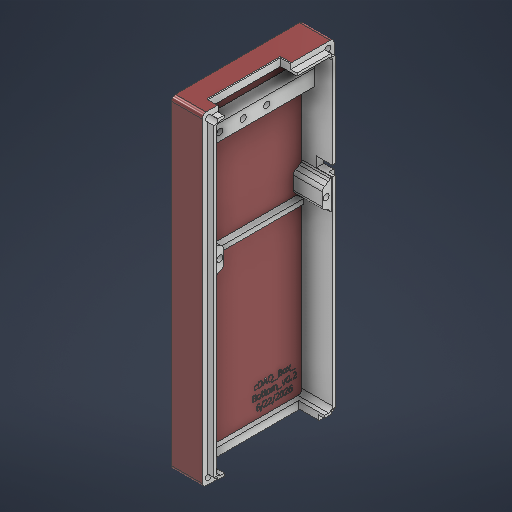
# Autodesk Inventor part: cDAQ_Box_Bottom_v0.2.2ipt
Saved by Autodesk Inventor 2027 (Build 310192000, 192)
## iProperties
Created: 2026-05-08
Part Number: cDAQ_Box_Bottom_v0.2.2ipt
Material: Generic
Document SubType Name: Modeling
Designer: giese
Density: 1 g/cm^3
Appearance: Default
Author: giese
Autodesk Inventor part; units mm, degrees
(part 1 of 2)
ref_plane "YZ Plane" through (0, 0, 0) normal (1, 0, 0) x (0, 1, 0)
ref_plane "XZ Plane" through (0, 0, 0) normal (0, 1, 0) x (-1, 0, 0)
ref_plane "XY Plane" through (0, 0, 0) normal (0, 0, 1) x (1, 0, 0)
sketch "Sketch1" plane through (0, 0, 0) normal (1, 0, 0) x (0, 1, 0)
  line L0 (37.5698, 55.7067) -> (-217.4462, 55.7067)
  line L1 (-217.4462, 55.7067) -> (-217.4462, -48.4333)
  line L2 (-217.4462, -48.4333) -> (37.5698, -48.4333)
  line L3 (37.5698, -48.4333) -> (37.5698, 55.7067)
  point P0 (0, 0)
  dimension "d0" = 104.14
  dimension "d1" = 255.016
  constraints: 8 end point, 2 parallel, 1 horizontal, 1 perpendicular
  measures "d0" distance of L2.end L0.start
  measures "d1" distance of L1.end L2.end
extrude "Extrusion1" add sketch "Sketch1" along normal blind 24.13
sketch "Sketch2" plane through (24.13, 0, 0) normal (1, 0, 0) x (0, 0, -1)
  line L0 (42.0833, 31.2198) -> (-49.3567, 31.2198)
  line L1 (-49.3567, 31.2198) -> (-49.3567, -211.0962)
  line L2 (-49.3567, -211.0962) -> (42.0833, -211.0962)
  line L3 (42.0833, -211.0962) -> (42.0833, 31.2198)
  line L4 (48.4333, 37.5698) -> (-55.7067, 37.5698) projected
  line L5 (-55.7067, 37.5698) -> (-55.7067, -217.4462) projected
  line L6 (-55.7067, -217.4462) -> (48.4333, -217.4462) projected
  line L7 (48.4333, -217.4462) -> (48.4333, 37.5698) projected
  point P0 (0, 0)
  dimension "d4" = 242.316
  dimension "d5" = 91.44
  dimension "d8" = 6.35
  dimension "d21" = 6.35
  dimension "d690" = 6.35
  dimension "d842" = 6.35
  constraints: 8 end point, 2 parallel, 1 horizontal, 1 perpendicular
  measures "d4" distance of L2.end L0.start
  measures "d5" distance of L0.start L0.end
  measures "d8" distance between parallel lines of L0 L4
  measures "d21" distance between parallel lines of L5 L1
  measures "d690" distance between parallel lines of L6 L2
  measures "d842" distance between parallel lines of L7 L3
extrude "Extrusion2" cut sketch "Sketch2" against normal blind 19.05 contours L3 L2 L1 L0
sketch "Sketch3" plane through (0, 0, 0) normal (-1, 0, 0) x (0, 0, 1)
  circle A0 centre (-4.1509, 9.6298) radius 2.4005
  circle A1 centre (14.3479, 9.6298) radius 2.4005
  circle A2 centre (32.8467, 9.6298) radius 2.4005
  line L0 (-48.4333, -217.4462) -> (-48.4333, 37.5698) projected
  line L1 (-48.4333, 37.5698) -> (55.7067, 37.5698) projected
  line L2 (55.7067, 37.5698) -> (55.7067, -217.4462) projected
  line L3 (49.3567, 31.2198) -> (-42.0833, 31.2198) projected
  point P0 (0, 0)
  point P1 (-0.896, -23.7433)
  point P2 (-45.1848, 27.0137)
  dimension "d9" = 18.4988
  dimension "d10" = 4.801
  dimension "d11" = 4.801
  dimension "d12" = 18.4988
  dimension "d13" = 36.9976
  dimension "d18" = 22.86
  dimension "d22" = 4.801
  dimension "d58" = 27.94
  constraints: 3 centre point
  measures "d9" distance of A0.centre A1.centre
  measures "d10" diameter of A1
  measures "d11" diameter of A2
  measures "d12" distance of A1.centre A2.centre
  measures "d13" distance of A0.centre A2.centre
  measures "d18" distance from line of L2 A2.centre
  measures "d22" diameter of A0
  measures "d58" distance from line of L1 A2.centre
extrude "Extrusion3" cut sketch "Sketch3" against normal blind 5.08
sketch "Sketch5" plane through (0, -217.4462, -48.4333) normal (0, 0, -1) x (-1, 0, 0)
  line L0 (-27.2034, 165.862) -> (-16.51, 165.862)
  line L1 (-16.51, 165.862) -> (-16.51, 173.862)
  line L2 (-16.51, 173.862) -> (-27.2034, 173.862)
  line L3 (-27.2034, 173.862) -> (-27.2034, 165.862)
  line L4 (0, 255.016) -> (-24.13, 255.016) projected
  line L5 (0, 0) -> (0, 255.016) projected
  line L6 (-24.13, 0) -> (-24.13, 255.016) projected
  line L7 (0, 0) -> (-24.13, 0) projected
  point P0 (0, 217.4462)
  point P1 (-21.8567, 173.862)
  point P2 (-21.8567, 165.862)
  dimension "d28" = 10.6934
  dimension "d30" = 8
  dimension "d31" = 16.51
  dimension "d215" = 3.0734
  dimension "d1133" = 165.862
  constraints: 8 end point, 2 midpoint, 2 parallel, 1 horizontal, 1 perpendicular
  measures "d28" distance between parallel lines of L1 L3
  measures "d30" distance of point (-21.857, 173.862) point (-21.857, 165.862)
  measures "d31" distance between parallel lines of L5 L1
  measures "d215" distance between parallel lines of L6 L3
  measures "d1133" distance between parallel lines of L7 L0
extrude "Extrusion4" cut sketch "Sketch5" against normal blind 24.13 contours L3 L2 L6 L0 | L6 L2 L1 L0
sketch "Sketch6" plane through (0, -217.4462, -48.4333) normal (0, -1, 0) x (1, 0, 0)
  line L0 (24.08, 55.136) -> (16.08, 55.136)
  line L1 (16.08, 45.136) -> (24.08, 45.136)
  line L2 (0, 104.14) -> (0, 0) projected
  line L3 (29.63, 53.1359) -> (29.63, 47.136)
  line L4 (24.08, 55.136) -> (29.63, 53.1359)
  line L5 (29.63, 47.136) -> (24.08, 45.136)
  line L6 (0, 0) -> (24.13, 0) projected
  line L7 (24.13, 97.79) -> (24.13, 6.35) projected
  line L8 (24.13, 41.9134) -> (24.13, 37.4697)
  line L9 (16.08, 55.136) -> (8.636, 55.136)
  line L10 (8.636, 55.136) -> (8.636, 45.136)
  line L11 (8.636, 45.136) -> (21.16, 45.136)
  point P0 (0, 48.4333)
  point P1 (20.08, 55.136)
  point P2 (20.08, 45.136)
  point P3 (16.08, 50.136)
  dimension "d39" = 6
  dimension "d48" = 55.136
  dimension "d221" = 0
  dimension "d223" = 2
  dimension "d224" = 2
  dimension "d225" = 5.5
  dimension "d227" = 5.55
  dimension "d672" = 8.636
  constraints: 18 end point, 2 horizontal, 2 midpoint, 2 parallel, 2 point on line, 1 perpendicular, 1 vertical
  measures "d39" distance of L3.start L3.end
  measures "d48" distance between parallel lines of L6 L0
  measures "d221" horizontal distance of L0.start L1.end
  measures "d223" vertical distance of L3.end L1.end
  measures "d224" vertical distance of L0.start L3.start
  measures "d225" distance between parallel lines of L3 L7
  measures "d227" distance from line of L1.end L3
  measures "d672" distance between parallel lines of L2 L10
extrude "Extrusion5" [suppressed]
sketch "Sketch7" plane through (0, 37.5698, 55.7067) normal (0, 1, 0) x (1, 0, 0)
  line L0 (31.0134, 69.85) -> (16.002, 69.85)
  line L1 (16.002, 69.85) -> (16.002, 12.7)
  line L2 (16.002, 12.7) -> (31.0134, 12.7)
  line L3 (31.0134, 12.7) -> (31.0134, 69.85)
  line L4 (0, 0) -> (24.13, 0) projected
  line L5 (0, 104.14) -> (0, 0) projected
  line L6 (24.13, 104.14) -> (24.13, 0) projected
  point P0 (0, 55.7067)
  point P1 (24.13, 69.85)
  point P2 (24.13, 12.7)
  dimension "d52" = 12.7
  dimension "d55" = 16.002
  dimension "d56" = 15.0114
  dimension "d57" = 6.8834
  dimension "d1195" = 69.85
  constraints: 8 end point, 2 parallel, 1 horizontal, 1 perpendicular
  measures "d52" distance between parallel lines of L4 L2
  measures "d55" distance between parallel lines of L5 L1
  measures "d56" distance between parallel lines of L3 L1
  measures "d57" distance between parallel lines of L6 L3
  measures "d1195" distance between parallel lines of L4 L0
extrude "Extrusion6" cut sketch "Sketch7" against normal blind 7.62
fillet "Fillet1" radius 3.175 4 edges at (12.065, 37.5698, -48.4333) (12.065, 37.5698, 55.7067) (12.065, -217.4462, -48.4333) (12.065, -217.4462, 55.7067)
sketch "Sketch8" plane through (0, 0, 0) normal (-1, 0, 0) x (0, 0, 1)
  line L0 (-5.9225, 6.0992) -> (-2.3919, 6.0992)
  line L1 (-5.9225, 13.1604) -> (-2.3919, 13.1604)
  line L2 (-5.9225, 6.0992) -> (-7.9609, 9.6298)
  line L3 (-5.9225, 13.1604) -> (-7.9609, 9.6298)
  line L4 (-2.3919, 6.0992) -> (-0.3536, 9.6298)
  line L5 (-2.3919, 13.1604) -> (-0.3536, 9.6298)
  circle A0 centre (-4.1509, 9.6298) radius 2.4005 projected
  line L6 (12.5763, 6.0992) -> (16.1069, 6.0992)
  line L7 (12.5763, 13.1604) -> (16.1069, 13.1604)
  line L8 (12.5763, 6.0992) -> (10.5379, 9.6298)
  line L9 (12.5763, 13.1604) -> (10.5379, 9.6298)
  line L10 (16.1069, 6.0992) -> (18.1453, 9.6298)
  line L11 (16.1069, 13.1604) -> (18.1453, 9.6298)
  circle A1 centre (14.3479, 9.6298) radius 2.4005 projected
  line L12 (31.0751, 6.0992) -> (29.0367, 9.6298)
  line L13 (31.0751, 13.1604) -> (29.0367, 9.6298)
  line L14 (31.0751, 6.0992) -> (34.6057, 6.0992)
  line L15 (31.0751, 13.1604) -> (34.6057, 13.1604)
  line L16 (34.6057, 6.0992) -> (36.6441, 9.6298)
  line L17 (34.6057, 13.1604) -> (36.6441, 9.6298)
  circle A2 centre (32.8467, 9.6298) radius 2.4005 projected
  point P0 (-4.1572, 6.0992)
  point P1 (14.3416, 6.0992)
  point P2 (32.8404, 6.0992)
  point P3 (-7.9609, 9.6298)
  point P4 (-0.3536, 9.6298)
  point P5 (18.1453, 9.6298)
  point P6 (10.5379, 9.6298)
  point P7 (36.6441, 9.6298)
  point P8 (29.0367, 9.6298)
  dimension "d60" = 7.0612
  dimension "d61" = 120
  dimension "d62" = 120
  dimension "d63" = 120
  dimension "d64" = 120
  dimension "d65" = 3.5306
  dimension "d66" = 3.5306
  dimension "d67" = 3.5306
  dimension "d68" = 3.5306
  dimension "d69" = 3.5306
  dimension "d70" = 3.5306
  dimension "d71" = 0
  dimension "d72" = 7.6074
  dimension "d73" = 3.81
  dimension "d74" = 0
  dimension "d75" = 7.0612
  dimension "d76" = 120
  dimension "d77" = 120
  dimension "d78" = 120
  dimension "d79" = 120
  dimension "d80" = 3.5306
  dimension "d81" = 3.5306
  dimension "d82" = 3.5306
  dimension "d83" = 3.5306
  dimension "d84" = 3.5306
  dimension "d85" = 3.5306
  dimension "d86" = 0
  dimension "d87" = 7.6074
  dimension "d91" = 0
  dimension "d92" = 3.81
  dimension "d93" = 7.0612
  dimension "d94" = 120
  dimension "d95" = 120
  dimension "d96" = 120
  dimension "d97" = 120
  dimension "d98" = 3.5306
  dimension "d99" = 3.5306
  dimension "d100" = 3.5306
  dimension "d101" = 3.5306
  dimension "d102" = 3.5306
  dimension "d103" = 3.5306
  dimension "d104" = 0
  dimension "d105" = 7.6074
  dimension "d108" = 0
  dimension "d109" = 3.81
  constraints: 36 end point, 6 horizontal, 3 midpoint
  measures "d60" distance from line of point (-4.157, 6.099) L1
  measures "d61" angle of L0 L2
  measures "d62" angle of L1 L3
  measures "d63" angle of L4 L0
  measures "d64" angle of L5 L1
  measures "d65" distance of L0.start L0.end
  measures "d66" distance of L1.start L1.end
  measures "d67" vertical distance of L1.start L3.end
  measures "d68" vertical distance of L0.start L2.end
  measures "d69" vertical distance of L1.end L5.end
  measures "d70" vertical distance of L0.end L4.end
  measures "d71" horizontal distance of L0.start L1.start
  measures "d72" distance of L4.end L2.end
  measures "d73" distance of A0.centre L2.end
  measures "d74" vertical distance of A0.centre L4.end
  measures "d75" distance from line of point (14.342, 6.099) L7
  measures "d76" angle of L6 L8
  measures "d77" angle of L7 L9
  measures "d78" angle of L10 L6
  measures "d79" angle of L11 L7
  measures "d80" distance of L8.start L6.end
  measures "d81" distance of L9.start L7.end
  measures "d82" vertical distance of L9.start L9.end
  measures "d83" vertical distance of L8.start L8.end
  measures "d84" vertical distance of L7.end L11.end
  measures "d85" vertical distance of L6.end L10.end
  measures "d86" horizontal distance of L8.start L9.start
  measures "d87" distance of L10.end L8.end
  measures "d91" vertical distance of A1.centre L8.end
  measures "d92" distance of A1.centre L8.end
  measures "d93" distance from line of point (32.84, 6.099) L15
  measures "d94" angle of L14 L12
  measures "d95" angle of L15 L13
  measures "d96" angle of L16 L14
  measures "d97" angle of L17 L15
  measures "d98" distance of L12.start L16.start
  measures "d99" distance of L15.start L15.end
  measures "d100" vertical distance of L15.start L13.end
  measures "d101" vertical distance of L12.start L12.end
  measures "d102" vertical distance of L15.end L17.end
  measures "d103" vertical distance of L16.start L16.end
  measures "d104" horizontal distance of L12.start L15.start
  measures "d105" distance of L16.end L12.end
  measures "d108" vertical distance of A2.centre L12.end
  measures "d109" distance of A2.centre L12.end
extrude "Extrusion7" cut sketch "Sketch8" against normal blind 4 contours L2 L3 L1 L5 L4 L0 | A0 | L8 L9 L7 L11 L10 L6 | A1 | L12 L13 L15 L17 L16 L14 | A2
sketch "Sketch9" plane through (5.08, 0, 0) normal (1, 0, 0) x (0, 0, -1)
  arc A0 (24.8089, -180.8044) -> (19.3527, -180.8044) centre (22.0808, -178.3302) ccw
  line L0 (45.2583, 37.5698) -> (14.1433, 37.5698) projected
  line L1 (42.0833, 31.2198) -> (42.0833, -43.5842) projected
  arc A1 (20.1758, -185.9502) -> (23.9858, -185.9502) centre (22.0808, -185.9502) ccw
  line L2 (23.9858, -185.9502) -> (23.9858, -182.9374)
  line L3 (20.1758, -185.9502) -> (20.1758, -182.9374)
  arc A2 (24.8089, -180.8044) -> (23.9858, -182.9374) centre (27.1608, -182.9374) ccw
  arc A3 (20.1758, -182.9374) -> (19.3527, -180.8044) centre (17.0008, -182.9374) ccw
  arc A4 (-25.9911, -180.8044) -> (-31.4473, -180.8045) centre (-28.7192, -178.3302) ccw
  arc A5 (-30.6242, -185.9366) -> (-26.8142, -185.9502) centre (-28.7192, -185.9502) ccw
  line L4 (-26.8142, -185.9502) -> (-26.8142, -182.9374)
  line L5 (-30.6242, -185.9366) -> (-30.6242, -182.9374)
  arc A6 (-25.9911, -180.8044) -> (-26.8142, -182.9374) centre (-23.6392, -182.9374) ccw
  arc A7 (-30.6242, -182.9374) -> (-31.4473, -180.8045) centre (-33.7992, -182.9374) ccw
  line L6 (-43.0067, 37.5698) -> (-52.5317, 37.5698) projected
  line L7 (-49.3567, -211.0962) -> (-49.3567, 31.2198) projected
  point P0 (0, 0)
  point P1 (42.0833, -211.0962)
  point P2 (23.9858, -181.4823)
  point P3 (20.1758, -181.4823)
  point P4 (-26.8142, -181.4823)
  point P5 (-30.6242, -181.4823)
  point P6 (-49.3567, 31.2198)
  point P7 (-46.8167, -217.4462)
  dimension "d112" = 215.9
  dimension "d114" = 7.366
  dimension "d116" = 3.81
  dimension "d117" = 223.52
  dimension "d118" = 3.175
  dimension "d119" = 7.366
  dimension "d120" = 3.81
  dimension "d121" = 3.175
  dimension "d122" = 215.9
  dimension "d123" = 223.52
  dimension "d125" = 0
  dimension "d128" = 50.8
  dimension "d129" = 20.0025
  dimension "d130" = 0
  constraints: 20 point on circle, 8 centre point, 8 end point, 8 tangent, 4 point on line, 2 equal radius, 2 parallel, 2 vertical, 1 other
  measures "d112" distance from line of L0 A0.centre
  measures "d114" diameter of A0
  measures "d116" diameter of A1
  measures "d117" distance from line of L0 A1.centre
  measures "d118" radius of A2
  measures "d119" diameter of A4
  measures "d120" diameter of A5
  measures "d121" radius of A6
  measures "d122" distance from line of A4.centre L6
  measures "d123" distance from line of L6 A5.centre
  measures "d125" horizontal distance of A5.centre A4.centre
  measures "d128" distance of A5.centre A1.centre
  measures "d129" distance from line of L1 A0.centre
  measures "d130" horizontal distance of A0.centre A1.centre
extrude "Extrusion8" [suppressed]
sketch "Sketch10" plane through (24.13, 0, 0) normal (1, 0, 0) x (0, 0, -1)
  line L0 (-49.3567, 31.2198) -> (42.0833, 31.2198) projected
  line L1 (-49.3567, 31.2198) -> (42.0833, 31.2198)
  line L2 (42.0833, 33.2264) -> (-46.8167, 33.2264)
  line L3 (-46.8167, 33.2264) -> (-51.3633, 33.2264)
  line L4 (-51.3633, 33.2264) -> (-51.3633, -213.1028)
  line L5 (-51.3633, -213.1028) -> (44.0899, -213.1028)
  line L6 (44.0899, -213.1028) -> (44.0899, 33.2264)
  line L7 (44.0899, 33.2264) -> (41.9392, 33.2264)
  line L8 (42.0833, 31.2198) -> (42.0833, -43.5842) projected
  line L9 (-49.3567, -211.0962) -> (-49.3567, 31.2198) projected
  line L10 (42.0833, -211.0962) -> (-49.3567, -211.0962) projected
  line L11 (45.2583, 37.5698) -> (14.1433, 37.5698) projected
  line L12 (42.0833, 31.2198) -> (42.0833, -211.0962)
  line L13 (42.0833, -211.0962) -> (-49.3567, -211.0962)
  line L14 (-52.5317, -217.4462) -> (45.2583, -217.4462) projected
  line L15 (-49.3567, -211.0962) -> (-49.3567, 31.2198)
  line L16 (-49.3567, 31.2198) -> (42.0833, 31.2198)
  point P0 (-46.8167, -217.4462)
  dimension "d202" = 2.0066
  dimension "d203" = 2.0066
  dimension "d204" = 2.0066
  dimension "d205" = 2.0066
  dimension "d208" = 4.3434
  constraints: 22 end point, 5 perpendicular, 3 point on line, 2 parallel, 1 collinear, 1 horizontal, 1 other
  measures "d202" distance between parallel lines of L0 L2
  measures "d203" distance between parallel lines of L6 L8
  measures "d205" distance between parallel lines of L5 L10
  measures "d208" distance between parallel lines of L11 L2
extrude "Extrusion9" add sketch "Sketch10" along normal blind 5
fillet "Fillet2" radius 3.175 8 edges at (17.105, 31.2198, -42.0833) (17.105, 31.2198, 49.3567) (17.105, -211.0962, 49.3567) (17.105, -211.0962, -42.0833) (26.63, 33.2264, -44.0899) (26.63, 33.2264, 51.3633) (26.63, -213.1028, -44.0899) (26.63, -213.1028, 51.3633)
sketch "Sketch13" plane through (29.13, 0, 0) normal (1, 0, 0) x (0, 0, -1)
  arc A0 (44.0833, 30.0448) -> (40.9083, 33.2198) centre (40.9083, 30.0448) ccw projected
  arc A1 (-45.6417, 33.2198) -> (-48.8167, 30.0448) centre (-45.6417, 30.0448) ccw projected
  arc A2 (40.9083, -212.0802) -> (44.0833, -208.9052) centre (40.9083, -208.9052) ccw projected
  arc A3 (-48.8167, -208.9052) -> (-45.6417, -212.0802) centre (-45.6417, -208.9052) ccw projected
  line L0 (-43.0067, 37.5698) -> (-52.5317, 37.5698) projected
  line L1 (-55.7067, 34.3948) -> (-55.7067, -214.2712) projected
  line L2 (-52.5317, -217.4462) -> (45.2583, -217.4462) projected
  arc A4 (-48.8167, -208.9052) -> (-45.6417, -212.0802) centre (-45.6417, -208.9052) ccw projected
  circle A5 centre (-50.6267, -212.3662) radius 2.4005
  circle A6 centre (43.3533, -212.3662) radius 2.4005
  line L3 (48.4333, -214.2712) -> (48.4333, 34.3948) projected
  circle A7 centre (43.3533, 32.4898) radius 2.4005
  line L4 (45.2583, 37.5698) -> (14.1433, 37.5698) projected
  circle A8 centre (-50.6267, 32.4898) radius 2.4005
  arc A9 (41.4904, -28.6131) -> (38.3154, -25.4381) centre (38.3154, -28.6131) ccw
  circle A10 centre (38.2733, -64.0302) radius 2.4005
  circle A11 centre (-45.5467, -64.0302) radius 2.4005
  point P0 (0, 0)
  point P1 (-47.8868, 32.2898)
  point P2 (-47.8868, -211.1503)
  point P3 (-47.8868, -211.1503)
  point P4 (45.8404, -24.2631)
  point P5 (42.6654, -21.0881)
  dimension "d178" = 5.08
  dimension "d179" = 5.08
  dimension "d180" = 4.801
  dimension "d181" = 5.08
  dimension "d182" = 5.08
  dimension "d183" = 4.801
  dimension "d184" = 4.801
  dimension "d185" = 5.08
  dimension "d186" = 5.08
  dimension "d187" = 4.801
  dimension "d188" = 5.08
  dimension "d189" = 5.08
  dimension "d326" = 4.801
  dimension "d327" = 10.16
  dimension "d328" = 101.6
  dimension "d329" = 4.801
  dimension "d330" = 10.16
  dimension "d331" = 101.6
  constraints: 7 centre point, 5 point on circle
  measures "d178" distance from line of L1 A5.centre
  measures "d179" distance from line of L2 A5.centre
  measures "d180" diameter of A5
  measures "d181" distance from line of L2 A6.centre
  measures "d182" distance from line of L3 A6.centre
  measures "d183" diameter of A6
  measures "d184" diameter of A7
  measures "d185" distance from line of L3 A7.centre
  measures "d186" distance from line of L4 A7.centre
  measures "d187" diameter of A8
  measures "d188" distance from line of L0 A8.centre
  measures "d189" distance from line of L1 A8.centre
  measures "d326" diameter of A10
  measures "d327" distance from line of L3 A10.centre
  measures "d328" distance from line of A10.centre L4
  measures "d329" diameter of A11
  measures "d330" distance from line of L1 A11.centre
  measures "d331" distance from line of L0 A11.centre
extrude "Extrusion11" cut sketch "Sketch13" against normal blind 25.4
sketch "Sketch14" plane through (5.08, 0, 0) normal (1, 0, 0) x (0, 0, -1)
  line L0 (10.8408, -186.2545) -> (30.0575, -186.2545) construction
  line L1 (30.0575, -186.2545) -> (30.0575, -184.305) construction
  line L2 (30.0575, -184.305) -> (10.8408, -184.305) construction
  line L3 (10.8408, -184.305) -> (10.8408, -186.2545) construction
  spline S0 degree 2 poles (5.944, -191.0006) (5.5883, -191.0006) (4.9992, -190.782) (4.788, -190.5597) knots 0 0 0 1 2 2 2
  spline S1 degree 2 poles (4.788, -190.5597) (4.5768, -190.3411) (4.3434, -189.6668) (4.3434, -189.2148) knots 0 0 0 1 2 2 2
  spline S2 degree 2 poles (4.3434, -189.2148) (4.3434, -188.7628) (4.5842, -188.1033) (4.788, -187.881) knots 0 0 0 1 2 2 2
  spline S3 degree 2 poles (4.788, -187.881) (4.9918, -187.655) (5.5957, -187.4141) (5.944, -187.4141) knots 0 0 0 1 2 2 2
  spline S4 degree 2 poles (5.944, -187.4141) (6.2255, -187.4141) (6.7517, -187.5735) (6.9554, -187.6772) knots 0 0 0 1 2 2 2
  line L4 (6.9554, -187.6772) -> (6.9554, -188.3256)
  line L5 (6.9554, -188.3256) -> (6.9221, -188.3256)
  spline S5 degree 2 poles (6.9221, -188.3256) (6.8591, -188.2737) (6.6664, -188.1403) (6.5294, -188.0699) knots 0 0 0 1 2 2 2
  spline S6 degree 2 poles (6.5294, -188.0699) (6.4071, -188.0106) (6.081, -187.918) (5.9328, -187.918) knots 0 0 0 1 2 2 2
  spline S7 degree 2 poles (5.9328, -187.918) (5.4845, -187.918) (4.9399, -188.596) (4.9399, -189.2148) knots 0 0 0 1 2 2 2
  spline S8 degree 2 poles (4.9399, -189.2148) (4.9399, -189.8187) (5.466, -190.4967) (5.9328, -190.4967) knots 0 0 0 1 2 2 2
  spline S9 degree 2 poles (5.9328, -190.4967) (6.2144, -190.4967) (6.7257, -190.2633) (6.9221, -190.0818) knots 0 0 0 1 2 2 2
  line L6 (6.9221, -190.0818) -> (6.9554, -190.0818)
  line L7 (6.9554, -190.0818) -> (6.9554, -190.7301)
  spline S10 degree 2 poles (6.9554, -190.7301) (6.8702, -190.7709) (6.6109, -190.8857) (6.5071, -190.9117) knots 0 0 0 1 2 2 2
  spline S11 degree 2 poles (6.5071, -190.9117) (6.3589, -190.9561) (6.1255, -191.0006) (5.944, -191.0006) knots 0 0 0 1 2 2 2
  spline S12 degree 2 poles (11.131, -188.6405) (11.131, -189.2666) (10.6234, -190.2744) (10.1973, -190.556) knots 0 0 0 1 2 2 2
  spline S13 degree 2 poles (10.1973, -190.556) (9.8491, -190.7746) (9.134, -190.9228) (8.5782, -190.9228) knots 0 0 0 1 2 2 2
  line L8 (8.5782, -190.9228) -> (7.526, -190.9228)
  line L9 (7.526, -190.9228) -> (7.526, -186.3508)
  line L10 (7.526, -186.3508) -> (8.5671, -186.3508)
  spline S14 degree 2 poles (8.5671, -186.3508) (9.2118, -186.3508) (9.9454, -186.5435) (10.2047, -186.7139) knots 0 0 0 1 2 2 2
  spline S15 degree 2 poles (10.2047, -186.7139) (10.6456, -187.0066) (11.131, -187.9736) (11.131, -188.6405) knots 0 0 0 1 2 2 2
  spline S16 degree 2 poles (10.4974, -188.6331) (10.4974, -188.107) (10.1492, -187.3623) (9.8046, -187.1511) knots 0 0 0 1 2 2 2
  spline S17 degree 2 poles (9.8046, -187.1511) (9.5601, -187.0066) (9.008, -186.8769) (8.5968, -186.8769) knots 0 0 0 1 2 2 2
  line L11 (8.5968, -186.8769) -> (8.1336, -186.8769)
  line L12 (8.1336, -186.8769) -> (8.1336, -190.3967)
  line L13 (8.1336, -190.3967) -> (8.5968, -190.3967)
  spline S18 degree 2 poles (8.5968, -190.3967) (9.0006, -190.3967) (9.6119, -190.267) (9.8602, -190.0929) knots 0 0 0 1 2 2 2
  spline S19 degree 2 poles (9.8602, -190.0929) (10.1788, -189.878) (10.4974, -189.1666) (10.4974, -188.6331) knots 0 0 0 1 2 2 2
  line L14 (11.2977, -190.9228) -> (12.839, -186.3508)
  line L15 (12.839, -186.3508) -> (13.5874, -186.3508)
  line L16 (13.5874, -186.3508) -> (15.1287, -190.9228)
  line L17 (15.1287, -190.9228) -> (14.4877, -190.9228)
  line L18 (14.4877, -190.9228) -> (14.0728, -189.6446)
  line L19 (14.0728, -189.6446) -> (12.3277, -189.6446)
  line L20 (12.3277, -189.6446) -> (11.9128, -190.9228)
  line L21 (11.9128, -190.9228) -> (11.2977, -190.9228)
  line L22 (13.9061, -189.1259) -> (13.1984, -186.9732)
  line L23 (13.1984, -186.9732) -> (12.4944, -189.1259)
  line L24 (12.4944, -189.1259) -> (13.9061, -189.1259)
  spline S20 degree 2 poles (19.3599, -192.0417) (19.1931, -192.0825) (18.83, -192.1269) (18.6485, -192.1269) knots 0 0 0 1 2 2 2
  spline S21 degree 2 poles (18.6485, -192.1269) (18.1335, -192.1269) (17.4925, -191.5526) (17.4629, -191.0191) knots 0 0 0 1 2 2 2
  spline S22 degree 2 poles (17.4629, -191.0191) (17.4221, -191.0191) (17.3517, -191.0191) (17.3221, -191.0191) knots 0 0 0 1 2 2 2
  spline S23 degree 2 poles (17.3221, -191.0191) (16.859, -191.0191) (16.1142, -190.7042) (15.8475, -190.3967) knots 0 0 0 1 2 2 2
  spline S24 degree 2 poles (15.8475, -190.3967) (15.5844, -190.0929) (15.3028, -189.2037) (15.3028, -188.6405) knots 0 0 0 1 2 2 2
  spline S25 degree 2 poles (15.3028, -188.6405) (15.3028, -188.0625) (15.5881, -187.1881) (15.8512, -186.8769) knots 0 0 0 1 2 2 2
  spline S26 degree 2 poles (15.8512, -186.8769) (16.118, -186.5694) (16.8627, -186.2545) (17.3221, -186.2545) knots 0 0 0 1 2 2 2
  spline S27 degree 2 poles (17.3221, -186.2545) (17.7889, -186.2545) (18.5373, -186.5805) (18.7967, -186.8769) knots 0 0 0 1 2 2 2
  spline S28 degree 2 poles (18.7967, -186.8769) (19.056, -187.177) (19.345, -188.0699) (19.345, -188.6405) knots 0 0 0 1 2 2 2
  spline S29 degree 2 poles (19.345, -188.6405) (19.345, -189.5297) (18.6522, -190.6857) (18.0483, -190.8894) knots 0 0 0 1 2 2 2
  spline S30 degree 2 poles (18.0483, -190.8894) (18.0631, -191.0599) (18.152, -191.3341) (18.2224, -191.4119) knots 0 0 0 1 2 2 2
  spline S31 degree 2 poles (18.2224, -191.4119) (18.3076, -191.5082) (18.541, -191.5971) (18.7485, -191.5971) knots 0 0 0 1 2 2 2
  spline S32 degree 2 poles (18.7485, -191.5971) (18.8708, -191.5971) (19.2042, -191.5193) (19.2783, -191.4897) knots 0 0 0 1 2 2 2
  line L25 (19.2783, -191.4897) -> (19.3599, -191.4897)
  line L26 (19.3599, -191.4897) -> (19.3599, -192.0417)
  spline S33 degree 2 poles (18.7115, -188.6405) (18.7115, -188.1848) (18.5151, -187.4845) (18.3373, -187.2548) knots 0 0 0 1 2 2 2
  spline S34 degree 2 poles (18.3373, -187.2548) (18.1557, -187.0177) (17.6444, -186.7806) (17.3258, -186.7806) knots 0 0 0 1 2 2 2
  spline S35 degree 2 poles (17.3258, -186.7806) (16.996, -186.7806) (16.4996, -187.0103) (16.3106, -187.2548) knots 0 0 0 1 2 2 2
  spline S36 degree 2 poles (16.3106, -187.2548) (16.1291, -187.4882) (15.9364, -188.1959) (15.9364, -188.6405) knots 0 0 0 1 2 2 2
  spline S37 degree 2 poles (15.9364, -188.6405) (15.9364, -189.5408) (16.6922, -190.5004) (17.3258, -190.5004) knots 0 0 0 1 2 2 2
  spline S38 degree 2 poles (17.3258, -190.5004) (17.9594, -190.5004) (18.7115, -189.5408) (18.7115, -188.6405) knots 0 0 0 1 2 2 2
  line L27 (23.0278, -191.8416) -> (19.5006, -191.8416)
  line L28 (19.5006, -191.8416) -> (19.5006, -191.4452)
  line L29 (19.5006, -191.4452) -> (23.0278, -191.4452)
  line L30 (23.0278, -191.4452) -> (23.0278, -191.8416)
  spline S39 degree 2 poles (26.5439, -189.5186) (26.5439, -189.8595) (26.2845, -190.3819) (26.0696, -190.5523) knots 0 0 0 1 2 2 2
  spline S40 degree 2 poles (26.0696, -190.5523) (25.8103, -190.7524) (25.2212, -190.9228) (24.7544, -190.9228) knots 0 0 0 1 2 2 2
  line L31 (24.7544, -190.9228) -> (23.4428, -190.9228)
  line L32 (23.4428, -190.9228) -> (23.4428, -186.3508)
  line L33 (23.4428, -186.3508) -> (24.6543, -186.3508)
  spline S41 degree 2 poles (24.6543, -186.3508) (25.1434, -186.3508) (25.6325, -186.4138) (25.8548, -186.536) knots 0 0 0 1 2 2 2
  spline S42 degree 2 poles (25.8548, -186.536) (26.103, -186.6657) (26.329, -187.0918) (26.329, -187.3808) knots 0 0 0 1 2 2 2
  spline S43 degree 2 poles (26.329, -187.3808) (26.329, -187.7031) (25.9881, -188.2144) (25.688, -188.3589) knots 0 0 0 1 2 2 2
  line L34 (25.688, -188.3589) -> (25.688, -188.3811)
  spline S44 degree 2 poles (25.688, -188.3811) (26.0956, -188.4923) (26.5439, -189.0814) (26.5439, -189.5186) knots 0 0 0 1 2 2 2
  spline S45 degree 2 poles (25.9103, -189.5445) (25.9103, -189.2852) (25.7621, -188.9517) (25.5398, -188.8332) knots 0 0 0 1 2 2 2
  spline S46 degree 2 poles (25.5398, -188.8332) (25.3953, -188.7591) (25.0545, -188.7146) (24.7395, -188.7146) knots 0 0 0 1 2 2 2
  line L35 (24.7395, -188.7146) -> (24.0504, -188.7146)
  line L36 (24.0504, -188.7146) -> (24.0504, -190.4041)
  line L37 (24.0504, -190.4041) -> (24.5432, -190.4041)
  spline S47 degree 2 poles (24.5432, -190.4041) (24.9433, -190.4041) (25.4027, -190.33) (25.5806, -190.2114) knots 0 0 0 1 2 2 2
  spline S48 degree 2 poles (25.5806, -190.2114) (25.751, -190.0892) (25.9103, -189.7854) (25.9103, -189.5445) knots 0 0 0 1 2 2 2
  spline S49 degree 2 poles (25.6954, -187.466) (25.6954, -187.303) (25.5843, -187.0585) (25.462, -186.9881) knots 0 0 0 1 2 2 2
  spline S50 degree 2 poles (25.462, -186.9881) (25.3138, -186.9065) (24.9544, -186.8695) (24.6321, -186.8695) knots 0 0 0 1 2 2 2
  line L38 (24.6321, -186.8695) -> (24.0504, -186.8695)
  line L39 (24.0504, -186.8695) -> (24.0504, -188.207)
  line L40 (24.0504, -188.207) -> (24.7395, -188.207)
  spline S51 degree 2 poles (24.7395, -188.207) (25.0248, -188.207) (25.2953, -188.1477) (25.4398, -188.0551) knots 0 0 0 1 2 2 2
  spline S52 degree 2 poles (25.4398, -188.0551) (25.5806, -187.9662) (25.6954, -187.6809) (25.6954, -187.466) knots 0 0 0 1 2 2 2
  spline S53 degree 2 poles (29.9229, -189.2074) (29.9229, -190.0743) (29.0892, -191.0191) (28.3927, -191.0191) knots 0 0 0 1 2 2 2
  spline S54 degree 2 poles (28.3927, -191.0191) (27.6776, -191.0191) (26.8588, -190.0447) (26.8588, -189.2074) knots 0 0 0 1 2 2 2
  spline S55 degree 2 poles (26.8588, -189.2074) (26.8588, -188.3478) (27.7036, -187.3956) (28.3927, -187.3956) knots 0 0 0 1 2 2 2
  spline S56 degree 2 poles (28.3927, -187.3956) (29.0892, -187.3956) (29.9229, -188.3441) (29.9229, -189.2074) knots 0 0 0 1 2 2 2
  spline S57 degree 2 poles (29.3264, -189.2074) (29.3264, -188.5405) (28.841, -187.8921) (28.3927, -187.8921) knots 0 0 0 1 2 2 2
  spline S58 degree 2 poles (28.3927, -187.8921) (27.9444, -187.8921) (27.4553, -188.5405) (27.4553, -189.2074) knots 0 0 0 1 2 2 2
  spline S59 degree 2 poles (27.4553, -189.2074) (27.4553, -189.8557) (27.9444, -190.5227) (28.3927, -190.5227) knots 0 0 0 1 2 2 2
  spline S60 degree 2 poles (28.3927, -190.5227) (28.8373, -190.5227) (29.3264, -189.8669) (29.3264, -189.2074) knots 0 0 0 1 2 2 2
  line L41 (33.1796, -190.9228) -> (32.4719, -190.9228)
  line L42 (32.4719, -190.9228) -> (31.6383, -189.6334)
  line L43 (31.6383, -189.6334) -> (30.7824, -190.9228)
  line L44 (30.7824, -190.9228) -> (30.1267, -190.9228)
  line L45 (30.1267, -190.9228) -> (31.316, -189.2222)
  line L46 (31.316, -189.2222) -> (30.1378, -187.4919)
  line L47 (30.1378, -187.4919) -> (30.8454, -187.4919)
  line L48 (30.8454, -187.4919) -> (31.6754, -188.7702)
  line L49 (31.6754, -188.7702) -> (32.5238, -187.4919)
  line L50 (32.5238, -187.4919) -> (33.1796, -187.4919)
  line L51 (33.1796, -187.4919) -> (31.9977, -189.1851)
  line L52 (31.9977, -189.1851) -> (33.1796, -190.9228)
  line L53 (36.6882, -191.8416) -> (33.1611, -191.8416)
  line L54 (33.1611, -191.8416) -> (33.1611, -191.4452)
  line L55 (33.1611, -191.4452) -> (36.6882, -191.4452)
  line L56 (36.6882, -191.4452) -> (36.6882, -191.8416)
  spline S61 degree 2 poles (6.3404, -197.0463) (6.3404, -197.3871) (6.081, -197.9095) (5.8662, -198.08) knots 0 0 0 1 2 2 2
  spline S62 degree 2 poles (5.8662, -198.08) (5.6068, -198.28) (5.0177, -198.4505) (4.5509, -198.4505) knots 0 0 0 1 2 2 2
  line L57 (4.5509, -198.4505) -> (3.2393, -198.4505)
  line L58 (3.2393, -198.4505) -> (3.2393, -193.8785)
  line L59 (3.2393, -193.8785) -> (4.4508, -193.8785)
  spline S63 degree 2 poles (4.4508, -193.8785) (4.9399, -193.8785) (5.429, -193.9415) (5.6513, -194.0637) knots 0 0 0 1 2 2 2
  spline S64 degree 2 poles (5.6513, -194.0637) (5.8995, -194.1934) (6.1255, -194.6195) (6.1255, -194.9085) knots 0 0 0 1 2 2 2
  spline S65 degree 2 poles (6.1255, -194.9085) (6.1255, -195.2308) (5.7846, -195.7421) (5.4845, -195.8866) knots 0 0 0 1 2 2 2
  line L60 (5.4845, -195.8866) -> (5.4845, -195.9088)
  spline S66 degree 2 poles (5.4845, -195.9088) (5.8921, -196.02) (6.3404, -196.6091) (6.3404, -197.0463) knots 0 0 0 1 2 2 2
  spline S67 degree 2 poles (5.7068, -197.0722) (5.7068, -196.8129) (5.5586, -196.4794) (5.3363, -196.3608) knots 0 0 0 1 2 2 2
  spline S68 degree 2 poles (5.3363, -196.3608) (5.1918, -196.2867) (4.851, -196.2423) (4.536, -196.2423) knots 0 0 0 1 2 2 2
  line L61 (4.536, -196.2423) -> (3.8469, -196.2423)
  line L62 (3.8469, -196.2423) -> (3.8469, -197.9318)
  line L63 (3.8469, -197.9318) -> (4.3397, -197.9318)
  spline S69 degree 2 poles (4.3397, -197.9318) (4.7398, -197.9318) (5.1992, -197.8577) (5.3771, -197.7391) knots 0 0 0 1 2 2 2
  spline S70 degree 2 poles (5.3771, -197.7391) (5.5475, -197.6168) (5.7068, -197.313) (5.7068, -197.0722) knots 0 0 0 1 2 2 2
  spline S71 degree 2 poles (5.4919, -194.9937) (5.4919, -194.8307) (5.3808, -194.5861) (5.2585, -194.5157) knots 0 0 0 1 2 2 2
  spline S72 degree 2 poles (5.2585, -194.5157) (5.1103, -194.4342) (4.7509, -194.3972) (4.4286, -194.3972) knots 0 0 0 1 2 2 2
  line L64 (4.4286, -194.3972) -> (3.8469, -194.3972)
  line L65 (3.8469, -194.3972) -> (3.8469, -195.7347)
  line L66 (3.8469, -195.7347) -> (4.536, -195.7347)
  spline S73 degree 2 poles (4.536, -195.7347) (4.8213, -195.7347) (5.0918, -195.6754) (5.2363, -195.5828) knots 0 0 0 1 2 2 2
  spline S74 degree 2 poles (5.2363, -195.5828) (5.3771, -195.4939) (5.4919, -195.2086) (5.4919, -194.9937) knots 0 0 0 1 2 2 2
  spline S75 degree 2 poles (9.7194, -196.735) (9.7194, -197.602) (8.8857, -198.5468) (8.1892, -198.5468) knots 0 0 0 1 2 2 2
  spline S76 degree 2 poles (8.1892, -198.5468) (7.4741, -198.5468) (6.6553, -197.5724) (6.6553, -196.735) knots 0 0 0 1 2 2 2
  spline S77 degree 2 poles (6.6553, -196.735) (6.6553, -195.8755) (7.5001, -194.9233) (8.1892, -194.9233) knots 0 0 0 1 2 2 2
  spline S78 degree 2 poles (8.1892, -194.9233) (8.8857, -194.9233) (9.7194, -195.8718) (9.7194, -196.735) knots 0 0 0 1 2 2 2
  spline S79 degree 2 poles (9.1229, -196.735) (9.1229, -196.0681) (8.6375, -195.4198) (8.1892, -195.4198) knots 0 0 0 1 2 2 2
  spline S80 degree 2 poles (8.1892, -195.4198) (7.7409, -195.4198) (7.2518, -196.0681) (7.2518, -196.735) knots 0 0 0 1 2 2 2
  spline S81 degree 2 poles (7.2518, -196.735) (7.2518, -197.3834) (7.7409, -198.0503) (8.1892, -198.0503) knots 0 0 0 1 2 2 2
  spline S82 degree 2 poles (8.1892, -198.0503) (8.6338, -198.0503) (9.1229, -197.3945) (9.1229, -196.735) knots 0 0 0 1 2 2 2
  spline S83 degree 2 poles (11.3496, -198.5172) (10.879, -198.5172) (10.3492, -197.9799) (10.3492, -197.3982) knots 0 0 0 1 2 2 2
  line L67 (10.3492, -197.3982) -> (10.3492, -195.4976)
  line L68 (10.3492, -195.4976) -> (9.9602, -195.4976)
  line L69 (9.9602, -195.4976) -> (9.9602, -195.0196)
  line L70 (9.9602, -195.0196) -> (10.3492, -195.0196)
  line L71 (10.3492, -195.0196) -> (10.3492, -194.0341)
  line L72 (10.3492, -194.0341) -> (10.9272, -194.0341)
  line L73 (10.9272, -194.0341) -> (10.9272, -195.0196)
  line L74 (10.9272, -195.0196) -> (11.9906, -195.0196)
  line L75 (11.9906, -195.0196) -> (11.9906, -195.4976)
  line L76 (11.9906, -195.4976) -> (10.9272, -195.4976)
  line L77 (10.9272, -195.4976) -> (10.9272, -197.1315)
  spline S84 degree 2 poles (10.9272, -197.1315) (10.9272, -197.3908) (10.9457, -197.6761) (11.0087, -197.7984) knots 0 0 0 1 2 2 2
  spline S85 degree 2 poles (11.0087, -197.7984) (11.0606, -197.9058) (11.294, -198.0133) (11.4941, -198.0133) knots 0 0 0 1 2 2 2
  spline S86 degree 2 poles (11.4941, -198.0133) (11.6349, -198.0133) (11.8979, -197.9281) (11.9572, -197.9021) knots 0 0 0 1 2 2 2
  line L78 (11.9572, -197.9021) -> (11.9906, -197.9021)
  line L79 (11.9906, -197.9021) -> (11.9906, -198.4208)
  spline S87 degree 2 poles (11.9906, -198.4208) (11.8275, -198.4653) (11.4941, -198.5172) (11.3496, -198.5172) knots 0 0 0 1 2 2 2
  spline S88 degree 2 poles (13.454, -198.5172) (12.9835, -198.5172) (12.4537, -197.9799) (12.4537, -197.3982) knots 0 0 0 1 2 2 2
  line L80 (12.4537, -197.3982) -> (12.4537, -195.4976)
  line L81 (12.4537, -195.4976) -> (12.0647, -195.4976)
  line L82 (12.0647, -195.4976) -> (12.0647, -195.0196)
  line L83 (12.0647, -195.0196) -> (12.4537, -195.0196)
  line L84 (12.4537, -195.0196) -> (12.4537, -194.0341)
  line L85 (12.4537, -194.0341) -> (13.0317, -194.0341)
  line L86 (13.0317, -194.0341) -> (13.0317, -195.0196)
  line L87 (13.0317, -195.0196) -> (14.095, -195.0196)
  line L88 (14.095, -195.0196) -> (14.095, -195.4976)
  line L89 (14.095, -195.4976) -> (13.0317, -195.4976)
  line L90 (13.0317, -195.4976) -> (13.0317, -197.1315)
  spline S89 degree 2 poles (13.0317, -197.1315) (13.0317, -197.3908) (13.0502, -197.6761) (13.1132, -197.7984) knots 0 0 0 1 2 2 2
  spline S90 degree 2 poles (13.1132, -197.7984) (13.165, -197.9058) (13.3985, -198.0133) (13.5985, -198.0133) knots 0 0 0 1 2 2 2
  spline S91 degree 2 poles (13.5985, -198.0133) (13.7393, -198.0133) (14.0024, -197.9281) (14.0617, -197.9021) knots 0 0 0 1 2 2 2
  line L91 (14.0617, -197.9021) -> (14.095, -197.9021)
  line L92 (14.095, -197.9021) -> (14.095, -198.4208)
  spline S92 degree 2 poles (14.095, -198.4208) (13.932, -198.4653) (13.5985, -198.5172) (13.454, -198.5172) knots 0 0 0 1 2 2 2
  spline S93 degree 2 poles (17.3406, -196.735) (17.3406, -197.602) (16.507, -198.5468) (15.8104, -198.5468) knots 0 0 0 1 2 2 2
  spline S94 degree 2 poles (15.8104, -198.5468) (15.0954, -198.5468) (14.2766, -197.5724) (14.2766, -196.735) knots 0 0 0 1 2 2 2
  spline S95 degree 2 poles (14.2766, -196.735) (14.2766, -195.8755) (15.1213, -194.9233) (15.8104, -194.9233) knots 0 0 0 1 2 2 2
  spline S96 degree 2 poles (15.8104, -194.9233) (16.507, -194.9233) (17.3406, -195.8718) (17.3406, -196.735) knots 0 0 0 1 2 2 2
  spline S97 degree 2 poles (16.7441, -196.735) (16.7441, -196.0681) (16.2587, -195.4198) (15.8104, -195.4198) knots 0 0 0 1 2 2 2
  spline S98 degree 2 poles (15.8104, -195.4198) (15.3621, -195.4198) (14.8731, -196.0681) (14.8731, -196.735) knots 0 0 0 1 2 2 2
  spline S99 degree 2 poles (14.8731, -196.735) (14.8731, -197.3834) (15.3621, -198.0503) (15.8104, -198.0503) knots 0 0 0 1 2 2 2
  spline S100 degree 2 poles (15.8104, -198.0503) (16.255, -198.0503) (16.7441, -197.3945) (16.7441, -196.735) knots 0 0 0 1 2 2 2
  line L93 (21.8237, -198.4505) -> (21.8237, -196.4646)
  spline S101 degree 2 poles (21.8237, -196.4646) (21.8237, -196.2275) (21.7866, -195.8236) (21.7274, -195.7125) knots 0 0 0 1 2 2 2
  spline S102 degree 2 poles (21.7274, -195.7125) (21.6681, -195.5902) (21.4421, -195.4716) (21.2457, -195.4716) knots 0 0 0 1 2 2 2
  spline S103 degree 2 poles (21.2457, -195.4716) (21.0679, -195.4716) (20.6603, -195.6902) (20.4454, -195.8977) knots 0 0 0 1 2 2 2
  spline S104 degree 2 poles (20.4454, -195.8977) (20.4491, -195.9496) (20.4565, -196.0941) (20.4565, -196.1904) knots 0 0 0 1 2 2 2
  line L94 (20.4565, -196.1904) -> (20.4565, -198.4505)
  line L95 (20.4565, -198.4505) -> (19.8786, -198.4505)
  line L96 (19.8786, -198.4505) -> (19.8786, -196.4646)
  spline S105 degree 2 poles (19.8786, -196.4646) (19.8786, -196.2275) (19.8415, -195.8236) (19.7822, -195.7125) knots 0 0 0 1 2 2 2
  spline S106 degree 2 poles (19.7822, -195.7125) (19.7229, -195.5902) (19.4969, -195.4716) (19.3006, -195.4716) knots 0 0 0 1 2 2 2
  spline S107 degree 2 poles (19.3006, -195.4716) (19.1153, -195.4716) (18.7041, -195.705) (18.5114, -195.8866) knots 0 0 0 1 2 2 2
  line L97 (18.5114, -195.8866) -> (18.5114, -198.4505)
  line L98 (18.5114, -198.4505) -> (17.9334, -198.4505)
  line L99 (17.9334, -198.4505) -> (17.9334, -195.0196)
  line L100 (17.9334, -195.0196) -> (18.5114, -195.0196)
  line L101 (18.5114, -195.0196) -> (18.5114, -195.3975)
  spline S108 degree 2 poles (18.5114, -195.3975) (18.7374, -195.1715) (19.182, -194.9233) (19.4488, -194.9233) knots 0 0 0 1 2 2 2
  spline S109 degree 2 poles (19.4488, -194.9233) (19.7526, -194.9233) (20.2231, -195.2012) (20.3454, -195.5161) knots 0 0 0 1 2 2 2
  spline S110 degree 2 poles (20.3454, -195.5161) (20.6084, -195.2234) (21.1049, -194.9233) (21.3939, -194.9233) knots 0 0 0 1 2 2 2
  spline S111 degree 2 poles (21.3939, -194.9233) (21.6162, -194.9233) (21.9793, -195.0604) (22.1127, -195.216) knots 0 0 0 1 2 2 2
  spline S112 degree 2 poles (22.1127, -195.216) (22.2498, -195.3716) (22.4017, -195.8384) (22.4017, -196.1904) knots 0 0 0 1 2 2 2
  line L102 (22.4017, -196.1904) -> (22.4017, -198.4505)
  line L103 (22.4017, -198.4505) -> (21.8237, -198.4505)
  line L104 (26.2734, -199.3693) -> (22.7462, -199.3693)
  line L105 (22.7462, -199.3693) -> (22.7462, -198.9729)
  line L106 (22.7462, -198.9729) -> (26.2734, -198.9729)
  line L107 (26.2734, -198.9729) -> (26.2734, -199.3693)
  line L108 (29.3375, -195.0196) -> (28.0444, -198.4505)
  line L109 (28.0444, -198.4505) -> (27.5257, -198.4505)
  line L110 (27.5257, -198.4505) -> (26.2438, -195.0196)
  line L111 (26.2438, -195.0196) -> (26.8699, -195.0196)
  line L112 (26.8699, -195.0196) -> (27.8073, -197.6613)
  line L113 (27.8073, -197.6613) -> (28.7373, -195.0196)
  line L114 (28.7373, -195.0196) -> (29.3375, -195.0196)
  spline S113 degree 2 poles (32.5349, -196.1645) (32.5349, -197.3945) (31.8198, -198.5468) (31.0751, -198.5468) knots 0 0 0 1 2 2 2
  spline S114 degree 2 poles (31.0751, -198.5468) (30.3193, -198.5468) (29.6117, -197.3723) (29.6117, -196.1682) knots 0 0 0 1 2 2 2
  spline S115 degree 2 poles (29.6117, -196.1682) (29.6117, -194.9307) (30.3267, -193.7858) (31.0751, -193.7858) knots 0 0 0 1 2 2 2
  spline S116 degree 2 poles (31.0751, -193.7858) (31.8273, -193.7858) (32.5349, -194.9715) (32.5349, -196.1645) knots 0 0 0 1 2 2 2
  spline S117 degree 2 poles (31.7495, -197.5576) (31.8384, -197.3316) (31.9125, -196.635) (31.9125, -196.1645) knots 0 0 0 1 2 2 2
  spline S118 degree 2 poles (31.9125, -196.1645) (31.9125, -195.6939) (31.8384, -195.0011) (31.7457, -194.7677) knots 0 0 0 1 2 2 2
  spline S119 degree 2 poles (31.7457, -194.7677) (31.6531, -194.5343) (31.3308, -194.2934) (31.0751, -194.2934) knots 0 0 0 1 2 2 2
  spline S120 degree 2 poles (31.0751, -194.2934) (30.8195, -194.2934) (30.4897, -194.5343) (30.3934, -194.7751) knots 0 0 0 1 2 2 2
  spline S121 degree 2 poles (30.3934, -194.7751) (30.3008, -195.0085) (30.2341, -195.7199) (30.2341, -196.1682) knots 0 0 0 1 2 2 2
  spline S122 degree 2 poles (30.2341, -196.1682) (30.2341, -196.6498) (30.2934, -197.2945) (30.3897, -197.5464) knots 0 0 0 1 2 2 2
  spline S123 degree 2 poles (30.3897, -197.5464) (30.4786, -197.7836) (30.8084, -198.0392) (31.0751, -198.0392) knots 0 0 0 1 2 2 2
  spline S124 degree 2 poles (31.0751, -198.0392) (31.3271, -198.0392) (31.6568, -197.7984) (31.7495, -197.5576) knots 0 0 0 1 2 2 2
  line L115 (34.1021, -198.4505) -> (33.3685, -198.4505)
  line L116 (33.3685, -198.4505) -> (33.3685, -197.5761)
  line L117 (33.3685, -197.5761) -> (34.1021, -197.5761)
  line L118 (34.1021, -197.5761) -> (34.1021, -198.4505)
  line L119 (37.8442, -198.4505) -> (35.0247, -198.4505)
  line L120 (35.0247, -198.4505) -> (35.0247, -197.8021)
  spline S125 degree 2 poles (35.0247, -197.8021) (35.3285, -197.5168) (35.8694, -196.987) (36.1288, -196.7017) knots 0 0 0 1 2 2 2
  spline S126 degree 2 poles (36.1288, -196.7017) (36.6512, -196.1274) (37.0328, -195.4383) (37.0328, -195.0715) knots 0 0 0 1 2 2 2
  spline S127 degree 2 poles (37.0328, -195.0715) (37.0328, -194.8788) (36.9143, -194.5898) (36.8068, -194.4972) knots 0 0 0 1 2 2 2
  spline S128 degree 2 poles (36.8068, -194.4972) (36.6994, -194.4046) (36.4178, -194.312) (36.2474, -194.312) knots 0 0 0 1 2 2 2
  spline S129 degree 2 poles (36.2474, -194.312) (36.0843, -194.312) (35.7509, -194.3935) (35.599, -194.4565) knots 0 0 0 1 2 2 2
  spline S130 degree 2 poles (35.599, -194.4565) (35.4693, -194.5083) (35.2285, -194.6565) (35.1544, -194.7084) knots 0 0 0 1 2 2 2
  line L121 (35.1544, -194.7084) -> (35.121, -194.7084)
  line L122 (35.121, -194.7084) -> (35.121, -194.0563)
  spline S131 degree 2 poles (35.121, -194.0563) (35.31, -193.9637) (35.988, -193.7821) (36.2918, -193.7821) knots 0 0 0 1 2 2 2
  spline S132 degree 2 poles (36.2918, -193.7821) (36.9328, -193.7821) (37.6553, -194.4602) (37.6553, -195.0381) knots 0 0 0 1 2 2 2
  spline S133 degree 2 poles (37.6553, -195.0381) (37.6553, -195.3086) (37.5293, -195.7606) (37.4181, -195.9533) knots 0 0 0 1 2 2 2
  spline S134 degree 2 poles (37.4181, -195.9533) (37.307, -196.1534) (36.9847, -196.5461) (36.8068, -196.735) knots 0 0 0 1 2 2 2
  spline S135 degree 2 poles (36.8068, -196.735) (36.5178, -197.05) (35.8102, -197.7243) (35.599, -197.9207) knots 0 0 0 1 2 2 2
  line L123 (35.599, -197.9207) -> (37.8442, -197.9207)
  line L124 (37.8442, -197.9207) -> (37.8442, -198.4505)
  spline S136 degree 2 poles (9.26, -204.4961) (9.26, -204.8481) (9.0265, -205.4446) (8.8302, -205.6447) knots 0 0 0 1 2 2 2
  spline S137 degree 2 poles (8.8302, -205.6447) (8.6264, -205.8559) (8.1151, -206.0745) (7.8076, -206.0745) knots 0 0 0 1 2 2 2
  spline S138 degree 2 poles (7.8076, -206.0745) (7.5001, -206.0745) (6.9925, -205.867) (6.7998, -205.6595) knots 0 0 0 1 2 2 2
  spline S139 degree 2 poles (6.7998, -205.6595) (6.5627, -205.4113) (6.2959, -204.5777) (6.2959, -203.97) knots 0 0 0 1 2 2 2
  spline S140 degree 2 poles (6.2959, -203.97) (6.2959, -203.3735) (6.5405, -202.4139) (6.7961, -202.0582) knots 0 0 0 1 2 2 2
  spline S141 degree 2 poles (6.7961, -202.0582) (7.0443, -201.71) (7.8298, -201.3209) (8.3448, -201.3209) knots 0 0 0 1 2 2 2
  spline S142 degree 2 poles (8.3448, -201.3209) (8.4967, -201.3209) (8.7635, -201.3506) (8.8635, -201.3839) knots 0 0 0 1 2 2 2
  line L125 (8.8635, -201.3839) -> (8.8635, -201.973)
  line L126 (8.8635, -201.973) -> (8.8376, -201.973)
  spline S143 degree 2 poles (8.8376, -201.973) (8.7524, -201.9286) (8.4411, -201.8508) (8.2633, -201.8508) knots 0 0 0 1 2 2 2
  spline S144 degree 2 poles (8.2633, -201.8508) (7.6927, -201.8508) (6.9925, -202.6214) (6.9258, -203.3772) knots 0 0 0 1 2 2 2
  spline S145 degree 2 poles (6.9258, -203.3772) (7.1444, -203.2253) (7.6038, -203.0586) (7.878, -203.0586) knots 0 0 0 1 2 2 2
  spline S146 degree 2 poles (7.878, -203.0586) (8.1447, -203.0586) (8.5449, -203.166) (8.7635, -203.3291) knots 0 0 0 1 2 2 2
  spline S147 degree 2 poles (8.7635, -203.3291) (9.0154, -203.518) (9.26, -204.1034) (9.26, -204.4961) knots 0 0 0 1 2 2 2
  spline S148 degree 2 poles (8.6375, -204.5221) (8.6375, -204.2405) (8.4893, -203.8589) (8.3263, -203.7255) knots 0 0 0 1 2 2 2
  spline S149 degree 2 poles (8.3263, -203.7255) (8.204, -203.6292) (7.9002, -203.5662) (7.7409, -203.5662) knots 0 0 0 1 2 2 2
  spline S150 degree 2 poles (7.7409, -203.5662) (7.526, -203.5662) (7.1222, -203.6959) (6.9258, -203.8181) knots 0 0 0 1 2 2 2
  spline S151 degree 2 poles (6.9258, -203.8181) (6.9221, -203.8848) (6.9147, -204.0108) (6.9147, -204.1071) knots 0 0 0 1 2 2 2
  spline S152 degree 2 poles (6.9147, -204.1071) (6.9147, -204.5814) (7.0999, -205.163) (7.2407, -205.315) knots 0 0 0 1 2 2 2
  spline S153 degree 2 poles (7.2407, -205.315) (7.3704, -205.4594) (7.652, -205.5743) (7.8113, -205.5743) knots 0 0 0 1 2 2 2
  spline S154 degree 2 poles (7.8113, -205.5743) (8.1818, -205.5743) (8.6375, -205.0482) (8.6375, -204.5221) knots 0 0 0 1 2 2 2
  line L127 (11.7016, -201.2024) -> (9.912, -206.9711)
  line L128 (9.912, -206.9711) -> (9.3933, -206.9711)
  line L129 (9.3933, -206.9711) -> (11.1755, -201.2024)
  line L130 (11.1755, -201.2024) -> (11.7016, -201.2024)
  line L131 (15.025, -205.9782) -> (12.2054, -205.9782)
  line L132 (12.2054, -205.9782) -> (12.2054, -205.3298)
  spline S155 degree 2 poles (12.2054, -205.3298) (12.5093, -205.0445) (13.0502, -204.5147) (13.3095, -204.2294) knots 0 0 0 1 2 2 2
  spline S156 degree 2 poles (13.3095, -204.2294) (13.832, -203.6551) (14.2136, -202.966) (14.2136, -202.5992) knots 0 0 0 1 2 2 2
  spline S157 degree 2 poles (14.2136, -202.5992) (14.2136, -202.4065) (14.095, -202.1175) (13.9876, -202.0249) knots 0 0 0 1 2 2 2
  spline S158 degree 2 poles (13.9876, -202.0249) (13.8801, -201.9323) (13.5985, -201.8396) (13.4281, -201.8396) knots 0 0 0 1 2 2 2
  spline S159 degree 2 poles (13.4281, -201.8396) (13.2651, -201.8396) (12.9316, -201.9211) (12.7797, -201.9841) knots 0 0 0 1 2 2 2
  spline S160 degree 2 poles (12.7797, -201.9841) (12.6501, -202.036) (12.4092, -202.1842) (12.3351, -202.2361) knots 0 0 0 1 2 2 2
  line L133 (12.3351, -202.2361) -> (12.3018, -202.2361)
  line L134 (12.3018, -202.2361) -> (12.3018, -201.584)
  spline S161 degree 2 poles (12.3018, -201.584) (12.4907, -201.4914) (13.1688, -201.3098) (13.4726, -201.3098) knots 0 0 0 1 2 2 2
  spline S162 degree 2 poles (13.4726, -201.3098) (14.1135, -201.3098) (14.836, -201.9878) (14.836, -202.5658) knots 0 0 0 1 2 2 2
  spline S163 degree 2 poles (14.836, -202.5658) (14.836, -202.8363) (14.71, -203.2883) (14.5989, -203.481) knots 0 0 0 1 2 2 2
  spline S164 degree 2 poles (14.5989, -203.481) (14.4877, -203.681) (14.1654, -204.0738) (13.9876, -204.2627) knots 0 0 0 1 2 2 2
  spline S165 degree 2 poles (13.9876, -204.2627) (13.6986, -204.5777) (12.9909, -205.252) (12.7797, -205.4483) knots 0 0 0 1 2 2 2
  line L135 (12.7797, -205.4483) -> (15.025, -205.4483)
  line L136 (15.025, -205.4483) -> (15.025, -205.9782)
  line L137 (18.4558, -205.9782) -> (15.6363, -205.9782)
  line L138 (15.6363, -205.9782) -> (15.6363, -205.3298)
  spline S166 degree 2 poles (15.6363, -205.3298) (15.9401, -205.0445) (16.481, -204.5147) (16.7404, -204.2294) knots 0 0 0 1 2 2 2
  spline S167 degree 2 poles (16.7404, -204.2294) (17.2628, -203.6551) (17.6444, -202.966) (17.6444, -202.5992) knots 0 0 0 1 2 2 2
  spline S168 degree 2 poles (17.6444, -202.5992) (17.6444, -202.4065) (17.5259, -202.1175) (17.4184, -202.0249) knots 0 0 0 1 2 2 2
  spline S169 degree 2 poles (17.4184, -202.0249) (17.311, -201.9323) (17.0294, -201.8396) (16.859, -201.8396) knots 0 0 0 1 2 2 2
  spline S170 degree 2 poles (16.859, -201.8396) (16.6959, -201.8396) (16.3625, -201.9211) (16.2106, -201.9841) knots 0 0 0 1 2 2 2
  spline S171 degree 2 poles (16.2106, -201.9841) (16.0809, -202.036) (15.8401, -202.1842) (15.766, -202.2361) knots 0 0 0 1 2 2 2
  line L139 (15.766, -202.2361) -> (15.7326, -202.2361)
  line L140 (15.7326, -202.2361) -> (15.7326, -201.584)
  spline S172 degree 2 poles (15.7326, -201.584) (15.9216, -201.4914) (16.5996, -201.3098) (16.9034, -201.3098) knots 0 0 0 1 2 2 2